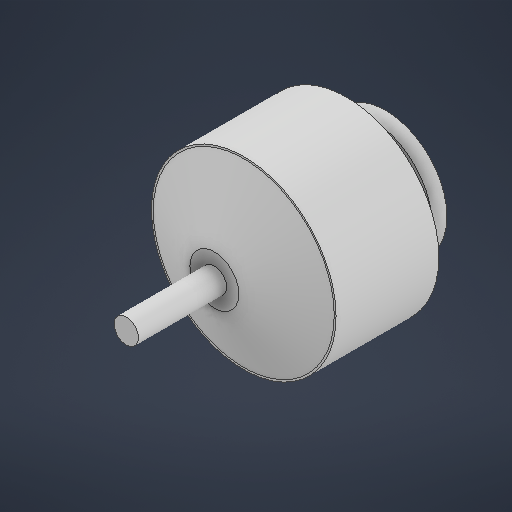
# Autodesk Inventor part: Двигатель 3115
Saved by Autodesk Inventor 2026 (Build 300175000, 175)
## iProperties
Created: 2025-08-20
Part Number: Двигатель 3115
Material: Типовые
Document SubType Name: Modeling
Designer: seraf
Density: 1 g/cm^3
Appearance: По умолчанию
Author: seraf
Autodesk Inventor part; units mm, degrees
ref_plane "YZ Plane" through (0, 0, 0) normal (1, 0, 0) x (0, 1, 0)
ref_plane "XZ Plane" through (0, 0, 0) normal (0, 1, 0) x (-1, 0, 0)
ref_plane "XY Plane" through (0, 0, 0) normal (0, 0, 1) x (1, 0, 0)
sketch "Эскиз1" plane through (0, 0, 0) normal (0, 0, 1) x (1, 0, 0)
  circle A0 centre (0, 0) radius 12.5
  dimension "d0" = 25
  constraints: 1 centre point, 1 coincident
  measures "d0" diameter of A0
extrude "Выдавливание1" add sketch "Эскиз1" along normal blind 3
sketch "Эскиз2" plane through (0, 0, 3) normal (0, 0, 1) x (1, 0, 0)
  circle A0 centre (0, 0) radius 7.5
  dimension "d3" = 15
  constraints: 1 centre point, 1 coincident
  measures "d3" diameter of A0
extrude "Выдавливание2" add sketch "Эскиз2" along normal blind 5
sketch "Эскиз3" plane through (0, 0, 8) normal (0, 0, 1) x (1, 0, 0)
  circle A0 centre (0, 0) radius 18.85
  dimension "d6" = 37.7
  constraints: 1 centre point, 1 coincident
  measures "d6" diameter of A0
extrude "Выдавливание3" add sketch "Эскиз3" along normal blind 21
sketch "Эскиз4" plane through (0, 0, 29) normal (0, 0, 1) x (1, 0, 0)
  circle A0 centre (0, 0) radius 5
  dimension "d9" = 10
  constraints: 1 centre point, 1 coincident
  measures "d9" diameter of A0
extrude "Выдавливание4" add sketch "Эскиз4" along normal blind 6
chamfer "Фаска1" distance 6 angle 66 1 edges at (-5, 0, 29) measured on face at (4.9353, -0.8021, 33)
sketch "Эскиз5" plane through (0, 0, 35) normal (0, 0, 1) x (1, 0, 0)
  circle A0 centre (0, 0) radius 2.5
  dimension "d15" = 5
  constraints: 1 centre point, 1 coincident
  measures "d15" diameter of A0
extrude "Выдавливание5" add sketch "Эскиз5" along normal blind 18
sketch "Эскиз6" plane through (0, 0, 0) normal (0, 0, -1) x (-1, 0, 0)
  circle A0 centre (0, 0) radius 9.5 construction
  circle A1 centre (0, 0) radius 12.5 construction
  line L0 (6.7175, -6.7175) -> (-6.7175, -6.7175) construction
  line L1 (-6.7175, -6.7175) -> (-6.7175, 6.7175) construction
  line L2 (-6.7175, 6.7175) -> (6.7175, 6.7175) construction
  line L3 (6.7175, 6.7175) -> (6.7175, -6.7175) construction
  line L4 (6.7175, -6.7175) -> (-6.7175, 6.7175) construction
  line L5 (-6.7175, -6.7175) -> (6.7175, 6.7175) construction
  circle A2 centre (6.7175, -6.7175) radius 1.5
  circle A3 centre (-6.7175, -6.7175) radius 1.5
  circle A4 centre (-6.7175, 6.7175) radius 1.5
  circle A5 centre (6.7175, 6.7175) radius 1.5
  dimension "d20" = 19
  dimension "d21" = 3
  dimension "d22" = 3
  dimension "d23" = 3
  dimension "d24" = 3
  constraints: 12 end point, 4 centre point, 4 coincident, 2 midpoint, 2 parallel, 2 perpendicular, 1 horizontal, 4 other
  measures "d21" diameter of A2
  measures "d22" diameter of A3
  measures "d23" diameter of A4
  measures "d24" diameter of A5
extrude "Выдавливание6" cut sketch "Эскиз6" against normal blind 5
